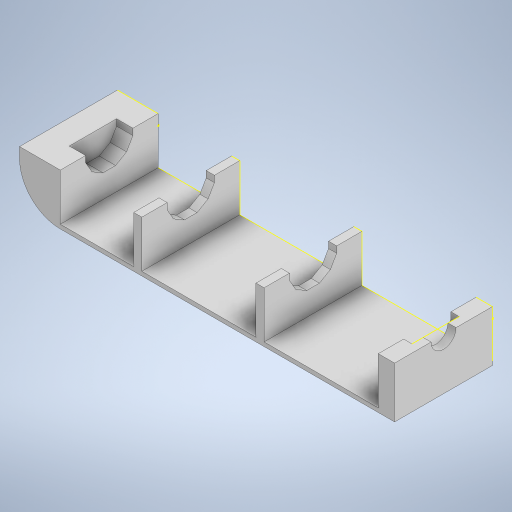
# Autodesk Inventor part: Support
Saved by Autodesk Inventor 2023 (Build 270158000, 158)
## iProperties
Created: 2024-07-10
Part Number: Support
Material: 일반
Document SubType Name: Modeling
Designer: ojs08
Density: 1 g/cm^3
Appearance: 기본값
Author: ojs08
Autodesk Inventor part; units mm, degrees
ref_plane "YZ Plane" through (0, 0, 0) normal (1, 0, 0) x (0, 1, 0)
ref_plane "XZ Plane" through (0, 0, 0) normal (0, 1, 0) x (-1, 0, 0)
ref_plane "XY Plane" through (0, 0, 0) normal (0, 0, 1) x (1, 0, 0)
sketch "스케치1" plane through (0, 0, 0) normal (0, 0, 1) x (1, 0, 0)
  arc A0 (-10, 0) -> (0, -10) centre (0, 0) ccw
  line L0 (-30.8853, 0) -> (100.8142, 0) projected
  line L1 (0, -14.9853) -> (0, 5.4142) projected
  line L2 (-10, 0) -> (-10, 2.5)
  line L3 (-10, 2.5) -> (0, 2.5)
  dimension "d1" = 20
  dimension "d2" = 2.5
  constraints: 4 end point, 3 point on line, 2 point on circle, 1 centre point, 1 coincident, 1 perpendicular, 1 vertical
  measures "d1" diameter of A0
  measures "d2" distance of L2.start L2.end
sketch "스케치2" plane through (0, 0, 0) normal (0, 0, 1) x (1, 0, 0)
  line L0 (0, -14.9853) -> (0, 5.4142) projected
  line L1 (-30.8853, 0) -> (100.8142, 0) projected
  line L2 (-10, 2.5) -> (0, 2.5) projected
  line L3 (0, 2.5) -> (0, -9)
  line L4 (0, -9) -> (18, -9)
  line L5 (18, -9) -> (18, 2.5)
  line L6 (18, 2.5) -> (20, 2.5)
  line L7 (20, 2.5) -> (20, -9)
  line L8 (20, -9) -> (48, -9)
  line L9 (48, -9) -> (48, 2.5)
  line L10 (48, 2.5) -> (50, 2.5)
  line L11 (50, 2.5) -> (50, -9)
  line L12 (50, -9) -> (78, -9)
  line L13 (78, -9) -> (78, 2.5)
  line L14 (78, 2.5) -> (82, 2.5)
  line L15 (82, 2.5) -> (82, -9)
  line L16 (82, -9) -> (82, -10)
  line L17 (0, -10) -> (82, -10)
  point P0 (0, 0)
  dimension "d3" = 11.5
  dimension "d4" = 18
  dimension "d5" = 2
  dimension "d6" = 11.5
  dimension "d7" = 28
  dimension "d8" = 2
  dimension "d9" = 11.5
  dimension "d10" = 28
  dimension "d11" = 4
  dimension "d12" = 11.5
  dimension "d13" = 1
  constraints: 30 end point, 9 perpendicular, 5 point on line, 4 horizontal, 1 vertical
  measures "d3" distance of L3.end L2.end
  measures "d4" distance of L3.end L4.end
  measures "d5" distance of L5.end L6.end
  measures "d6" distance of L6.end L7.end
  measures "d7" distance of L7.end L8.end
  measures "d8" distance of L9.end L10.end
  measures "d9" distance of L10.end L11.end
  measures "d10" distance of L11.end L12.end
  measures "d11" distance of L13.end L14.end
  measures "d12" distance of L14.end L15.end
  measures "d13" distance of L15.end L16.end
sketch "스케치3" plane through (0, 0, 0) normal (0, 0, 1) x (1, 0, 0)
  arc A0 (-10, 0) -> (0, -10) centre (0, 0) ccw projected
  line L0 (-10, 0) -> (-10, 2.5) projected
  line L1 (-10, 2.5) -> (0, 2.5) projected
  line L2 (0, -9) -> (18, -9) projected
  line L3 (0, -10) -> (82, -10) projected
  line L4 (18, -9) -> (18, 2.5) projected
  line L5 (18, 2.5) -> (20, 2.5) projected
  line L6 (20, 2.5) -> (20, -9) projected
  line L7 (20, -9) -> (48, -9) projected
  line L8 (48, -9) -> (48, 2.5) projected
  line L9 (50, 2.5) -> (50, -9) projected
  line L10 (48, 2.5) -> (50, 2.5) projected
  line L11 (50, -9) -> (78, -9) projected
  line L12 (78, -9) -> (78, 2.5) projected
  line L13 (78, 2.5) -> (82, 2.5) projected
  line L14 (82, 2.5) -> (82, -9) projected
extrude "돌출1" add sketch "스케치2" along normal blind 24 contours L0 L4 L5 L1 L7 L8 L9 L11 L12 L13 L15 L16 L17 | L5 L6 L7 L1 | L1 L13 L14 L15 | L9 L10 L11 L1
extrude "돌출2" add sketch "스케치1" along normal blind 24
sketch "스케치4" plane through (0, -9, 0) normal (1, 0, 0) x (0, 0, -1)
  point P0 (0, 9)
sketch "스케치5" plane through (0, -9, 0) normal (1, 0, 0) x (0, 0, -1)
  line L0 (-6.205, 11.5) -> (-6.205, 9.9472)
  line L1 (-6.205, 9.9472) -> (-7.7578, 7.2578)
  line L2 (-7.7578, 7.2578) -> (-10.4472, 5.705)
  line L3 (-10.4472, 5.705) -> (-13.5528, 5.705)
  line L4 (-13.5528, 5.705) -> (-16.2422, 7.2578)
  line L5 (-16.2422, 7.2578) -> (-17.795, 9.9472)
  line L6 (-17.795, 9.9472) -> (-17.795, 11.5)
  line L7 (0, 0) -> (-24, 0) projected
  line L8 (0, 11.5) -> (-24, 11.5) projected
  point P0 (0, 9)
  point P1 (-12, 11.5)
  point P2 (-12, 0)
  point P3 (-12, 11.5)
  dimension "d18" = 11.59
  constraints: 14 end point, 2 midpoint, 2 point on line, 1 coincident, 12 other
  measures "d18" distance of L6.end L0.start
extrude "돌출3" cut sketch "스케치5" against normal blind 4
sketch "스케치6" plane through (0, -9, 0) normal (1, 0, 0) x (0, 0, -1)
  line L0 (-13.5528, 5.705) -> (-16.2422, 7.2578) projected
  line L1 (-10.4472, 5.705) -> (-13.5528, 5.705) projected
  line L2 (-7.7578, 7.2578) -> (-10.4472, 5.705) projected
  line L3 (-6.205, 9.9472) -> (-7.7578, 7.2578) projected
  line L4 (-6.205, 11.5) -> (-6.205, 9.9472) projected
  line L5 (-17.795, 11.5) -> (-6.205, 11.5) projected
  line L6 (-17.795, 9.9472) -> (-17.795, 11.5) projected
  line L7 (-16.2422, 7.2578) -> (-17.795, 9.9472) projected
  point P0 (0, 9)
extrude "돌출4" cut sketch "스케치6" along normal blind 80
sketch "스케치7" plane through (82, -10, 0) normal (1, 0, 0) x (0, 0, -1)
  point P0 (0, 10)
sketch "스케치8" plane through (80, -9, 0) normal (-1, 0, 0) x (0, 0, 1)
  line L0 (6.205, 11.5) -> (17.795, 11.5) projected
  line L1 (10.4472, 5.705) -> (7.7578, 7.2578) projected
  line L2 (13.5528, 5.705) -> (10.4472, 5.705) projected
  line L3 (16.2422, 7.2578) -> (13.5528, 5.705) projected
  line L4 (17.795, 9.9472) -> (16.2422, 7.2578) projected
  line L5 (17.795, 11.5) -> (17.795, 9.9472) projected
  line L6 (6.205, 11.5) -> (17.795, 11.5) projected
  line L7 (6.205, 9.9472) -> (6.205, 11.5) projected
  line L8 (7.7578, 7.2578) -> (6.205, 9.9472) projected
  point P0 (0, 9)
sketch "스케치9" plane through (82, -10, 0) normal (1, 0, 0) x (0, 0, -1)
  arc A0 (-15.055, 12.5) -> (-8.945, 12.5) centre (-12, 12.5) ccw
  line L0 (0, 12.5) -> (-24, 12.5) projected
  point P0 (0, 10)
  constraints: 2 coincident, 2 point on circle, 2 point on line, 1 centre point, 1 midpoint
extrude "돌출5" cut sketch "스케치9" against normal up to surface (2 mm away)
